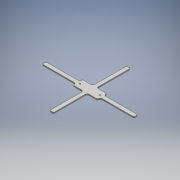
# Autodesk Inventor part: spin_light_tester
Saved by Autodesk Inventor 2016 (Build 200138000, 138)
## iProperties
Created: 2016-10-26
Part Number: spin_light_tester
Material: Generic
Document SubType Name: Modeling
Designer: rawrdong
Density: 1 g/cm^3
Appearance: Default
Author: rawrdong
Autodesk Inventor part; units mm, degrees
ref_plane "YZ Plane" through (0, 0, 0) normal (1, 0, 0) x (0, 1, 0)
ref_plane "XZ Plane" through (0, 0, 0) normal (0, 1, 0) x (-1, 0, 0)
ref_plane "XY Plane" through (0, 0, 0) normal (0, 0, 1) x (1, 0, 0)
sketch "Sketch1" plane through (0, 0, 0) normal (0, 0, 1) x (1, 0, 0)
  line L0 (-32.5, -12.5) -> (32.5, -12.5)
  line L1 (32.5, -12.5) -> (32.5, 12.5)
  line L2 (32.5, 12.5) -> (-32.5, 12.5)
  line L3 (-32.5, 12.5) -> (-32.5, -12.5)
  line L4 (-32.5, -12.5) -> (32.5, 12.5) construction
  line L5 (32.5, -12.5) -> (-32.5, 12.5) construction
  line L6 (32.5, 5) -> (122.5, 5)
  line L7 (122.5, 5) -> (122.5, -5)
  line L8 (122.5, -5) -> (32.5, -5)
  line L9 (-5, 12.5) -> (-5, 102.5)
  line L10 (-5, 102.5) -> (5, 102.5)
  line L11 (5, 102.5) -> (5, 12.5)
  line L12 (-32.5, 5) -> (-122.5, 5)
  line L13 (-122.5, 5) -> (-122.5, -5)
  line L14 (-122.5, -5) -> (-32.5, -5)
  line L15 (-5, -12.5) -> (-5, -102.5)
  line L16 (-5, -102.5) -> (5, -102.5)
  line L17 (5, -102.5) -> (5, -12.5)
  circle A0 centre (-26.6, 0) radius 1.6
  circle A1 centre (26.6, 0) radius 1.6
  line L18 (0, 0) -> (0, 12.5) construction
  line L19 (-26.6, 0) -> (26.6, 0) construction
  dimension "d0" = 90
  dimension "d1" = 53.2
  dimension "d2" = 10
  dimension "d3" = 3.2
  dimension "d4" = 65
  dimension "d5" = 25
  dimension "d6" = 90
  constraints: 40 end point, 14 point on line, 6 perpendicular, 4 equal length, 4 horizontal, 4 midpoint, 2 centre point, 2 horizontal alignment, 2 parallel, 2 vertical, 1 equal radius, 1 symmetric about line, 2 other
  measures "d0" distance of L10.end L11.end
  measures "d1" distance of L19.start L19.end
  measures "d2" distance of L6.end L7.end
  measures "d3" diameter of A0
  measures "d4" distance of L0.start L0.end
  measures "d5" distance of L0.end L1.end
  measures "d6" distance of L6.start L6.end
extrude "Extrusion1" add sketch "Sketch1" along normal blind 3
fillet "Fillet1" radius 2 12 edges at (32.5, 12.5, 1.5) (5, 102.5, 1.5) (-5, 102.5, 1.5) (-122.5, 5, 1.5) (-122.5, -5, 1.5) (-32.5, 12.5, 1.5) (-32.5, -12.5, 1.5) (-5, -102.5, 1.5) (5, -102.5, 1.5) (32.5, -12.5, 1.5) (122.5, -5, 1.5) (122.5, 5, 1.5)
fillet "Fillet1" radius 5 8 edges at (5, -12.5, 1.5) (-5, -12.5, 1.5) (32.5, -5, 1.5) (32.5, 5, 1.5) (5, 12.5, 1.5) (-5, 12.5, 1.5) (-32.5, -5, 1.5) (-32.5, 5, 1.5)
body "Solid1"
